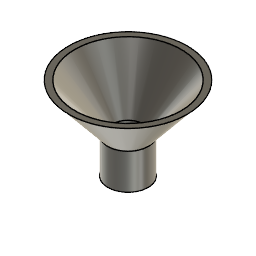
Water bottle funnel (Autodesk Fusion 360 design; units mm, degrees)
part number: 2026-08-03-12-30-00-447
Autodesk Fusion 360 part; units mm, degrees
sketch "Sketch1" plane through (0, 0, 0) normal (0, 0, 1) x (1, 0, 0)
  circle A0 centre (0, 0) radius 8.5
  dimension "d6" = 17
  constraint coincident A0.centre origin
  measures "d6" diameter of A0
extrude "Extrude1" add sketch "Sketch1" along normal blind 15
ref_plane "WorkPlane1" through (0, 0, 35) normal (0, 0, 1) x (1, 0, 0)
sketch "Sketch2" plane through (0, 0, 35) normal (0, 0, 1) x (1, 0, 0)
  circle A0 centre (0, 0) radius 25
  dimension "d10" = 50
  constraint coincident A0.centre origin
  measures "d10" diameter of A0
loft "Loft1" add profiles "Sketch2" section 1 section 2 face at (2.7075, 1.6235, 15)
shell "Shell1" thickness 2 removed faces 2 at (2.7075, 1.6235, 0) at (-6.7759, -1.242, 35)
equation "FH = 20 mm" comment "funnel height"
equation "TL = 15 mm" comment "Tube Length"
equation "WT = 2 mm" comment "Wall Thickness"
equation "LD = 50 mm" comment "Large Diameter"
equation "SD = 17 mm" comment "Small Diameter"
equation "d6 = SD"
equation "d7 = TL"
equation "d9 = FH"
equation "d10 = LD"
equation "d11 = WT"
